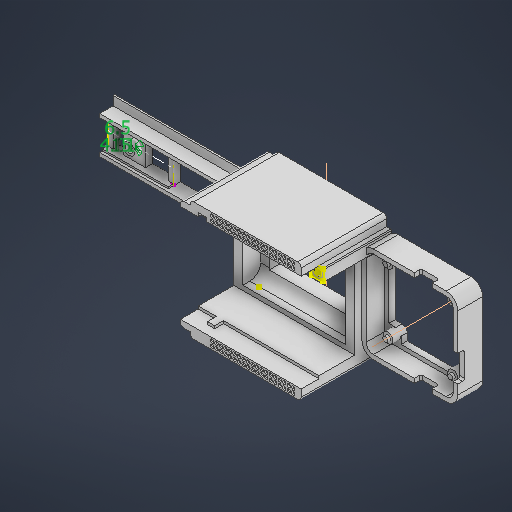
# Autodesk Inventor part: Base
Saved by Autodesk Inventor 2026 (Build 300175000, 175)
## iProperties
Created: 2026-08-27
Part Number: Base
Material: Generisch
Document SubType Name: Modeling
Designer: Fabian.Reifler
Density: 1 g/cm^3
Appearance: Vorgabe
Author: Fabian.Reifler
Autodesk Inventor part; units mm, degrees
sketch "Skizze1" plane through (0, 0, 0) normal (0, 0, 1) x (1, 0, 0)
  line L0 (-101.9645, 0) -> (106.7595, 0) construction
  line L1 (0, 139.1986) -> (0, -67.3687) construction
  line L2 (-143.7094, 0) -> (148.5043, 0) construction
  line L3 (0, -108.6821) -> (0, 180.5121) construction
  line L4 (-29, 23.45) -> (29, 23.45)
  line L5 (29, 23.45) -> (29, -23.45)
  line L6 (29, -23.45) -> (-29, -23.45)
  line L7 (-29, -23.45) -> (-29, 23.45)
  line L8 (-2.8134, 20.75) -> (4.8357, 20.75) construction
  line L9 (-2.8134, -20.75) -> (4.8357, -20.75) construction
  line L10 (-2.8134, 24.75) -> (4.8357, 24.75) construction
  line L11 (-2.8134, -24.75) -> (4.8357, -24.75) construction
  line L12 (-2.8134, 22.75) -> (5.1647, 22.75) construction
  circle A0 centre (0, 22.75) radius 2 construction
  circle A1 centre (0, -22.75) radius 2 construction
  line L13 (24, 18.45) -> (-24, 18.45)
  line L14 (-24, 18.45) -> (-24, -18.45)
  line L15 (-24, -18.45) -> (24, -18.45)
  line L16 (24, -18.45) -> (24, 18.45)
  line L17 (34, 28.45) -> (-34, 28.45)
  line L18 (-34, 28.45) -> (-34, -28.45)
  line L19 (-34, -28.45) -> (34, -28.45)
  line L20 (34, -28.45) -> (34, 28.45)
  line L21 (5, -40.2387) -> (5, 39.5986) construction
  line L22 (0, -22.75) -> (14.5212, -22.75) construction
  line L23 (0, 22.75) -> (17.4415, 22.75) construction
  point P0 (0, 0)
  point P1 (0, 24.75)
  point P2 (-1.8735, 23.45)
  point P3 (1.8735, 23.45)
  point P4 (5, 22.75)
  point P5 (5, -22.75)
  dimension "d0" = 58
  dimension "d1" = 46.9
  dimension "d2" = 41.5
  dimension "d3" = 4
  dimension "d4" = 5
  dimension "d5" = 5
  dimension "d79" = 10
  dimension "d104" = 5
  constraints: 44 end point, 10 point on line, 8 parallel, 7 horizontal, 4 perpendicular, 3 point on circle, 3 symmetric about line, 2 centre point, 2 collinear, 2 vertical, 1 coincident, 11 other
  measures "d0" distance of L4.start L4.end
  measures "d1" distance of L4.end L5.end
  measures "d2" distance between parallel lines of L9 L8
  measures "d3" distance between parallel lines of L10 L8
  measures "d4" distance between parallel lines of L4 L13
  measures "d5" distance between parallel lines of L4 L17
  measures "d79" diameter of L21 L3
  measures "d104" distance between parallel lines of L6 L15
extrude "Extrusion1" add sketch "Skizze1" along normal blind 8 contours L4 L5 L6 L7 | L16 L15 L14 L13 | L20 L19 L18 L17
extrude "Extrusion3" cut sketch "Skizze1" along normal through all contours L16 L15 L14 L13
hole "Bohrung1" at (5, -22.75, 0) at (5, 22.75, 0) direction (0, 0, 1) diameter 4.01 depth 6.5
sketch "Skizze2" plane through (0, 0, 8) normal (0, 0, 1) x (1, 0, 0)
  line L0 (29, 23.45) -> (29, -23.45) projected
  line L1 (29, -23.45) -> (-29, -23.45) projected
  line L2 (-29, 23.45) -> (29, 23.45) projected
  line L3 (-29, -23.45) -> (-29, 23.45) projected
  line L4 (-34, -28.45) -> (34, -28.45) projected
  line L5 (34, -28.45) -> (34, 28.45) projected
  line L6 (34, 28.45) -> (-34, 28.45) projected
  line L7 (-34, 28.45) -> (-34, -28.45) projected
  point P0 (0, 0)
extrude "Extrusion4" add sketch "Skizze2" along normal blind 10
fillet "Rundung1" radius 6 2 edges at (0, 23.45, 8) (0, -23.45, 8)
sketch "Skizze5" plane through (0, 0, 0) normal (0, 1, 0) x (-1, 0, 0)
  line L0 (-24, 8.0839) -> (24, 8.0839) projected
  line L1 (-31.8844, 48.0839) -> (73.7632, 48.0839)
  point P0 (0, 0)
  point P1 (0, 48.0839)
  dimension "d30" = 40
  constraints: 2 end point, 1 parallel, 1 point on line
  measures "d30" distance between parallel lines of L1 L0
ref_plane "Arbeitsebene6" through (0, 0, 48.0839) normal (0, 0, 1) x (1, 0, 0)
sketch "Skizze3" plane through (0, 0, 18) normal (0, 0, 1) x (1, 0, 0)
  line L0 (-34, 27.5) -> (34, 27.5)
  line L1 (34, 27.5) -> (34, -27.5)
  line L2 (34, -27.5) -> (-34, -27.5)
  line L3 (-34, -27.5) -> (-34, 27.5)
  line L4 (-95.3158, 0) -> (55.5526, 0) projected
  line L5 (0, -46.9) -> (0, 46.9) projected
  line L6 (-34, 27.5) -> (34, 27.5)
  line L7 (34, 27.5) -> (34, 33.5)
  line L8 (34, 33.5) -> (-34, 33.5)
  line L9 (-34, 33.5) -> (-34, 27.5)
  line L10 (-34, -27.5) -> (34, -27.5)
  line L11 (34, -27.5) -> (34, -33.5)
  line L12 (34, -33.5) -> (-34, -33.5)
  line L13 (-34, -33.5) -> (-34, -27.5)
  line L14 (34, -28.45) -> (34, 28.45) projected
  point P0 (0, 0)
  dimension "d22" = 55
  dimension "d24" = 6
  constraints: 24 end point, 4 parallel, 4 symmetric about line, 2 horizontal, 2 perpendicular, 1 collinear, 1 point on line, 2 other
  measures "d22" distance between parallel lines of L2 L0
  measures "d24" distance between parallel lines of L8 L0
extrude "Extrusion5" add sketch "Skizze3" along normal up to surface (30.0839 mm away) contours L9 L8 L5 L0 | L5 L8 L7 L0 | L2 L5 L12 L13 | L2 L11 L12 L5
sketch "Skizze4" plane through (0, 0, 18) normal (0, 0, -1) x (-1, 0, 0)
  line L0 (-34, 33.5) -> (34, 33.5) projected
  line L1 (34, 33.5) -> (34, 28.45) projected
  line L2 (-34, 28.45) -> (-34, 33.5) projected
  line L3 (-34, 28.45) -> (34, 28.45) projected
  line L4 (34, -33.5) -> (-34, -33.5) projected
  line L5 (34, -28.45) -> (34, -33.5) projected
  line L6 (-34, -33.5) -> (-34, -28.45) projected
  line L7 (34, -28.45) -> (-34, -28.45) projected
  point P0 (0, 0)
  point P1 (33.5, 28.45)
  point P2 (-33.5, 28.45)
  point P3 (33.5, -28.45)
  point P4 (-33.5, -28.45)
  constraints: 4 other
extrude "Extrusion6" add sketch "Skizze4" along normal up to surface (18 mm away)
fillet "Rundung2" radius 2 4 edges at (-34, -33.5, 24.042) (-34, 33.5, 24.042) (34, 33.5, 24.042) (34, -33.5, 24.042)
sketch "Skizze6" plane through (-34, 27.5, 48.0839) normal (0, 0, 1) x (1, 0, 0)
  line L0 (68, 0) -> (0, 0) projected
  line L1 (10, 0) -> (14.5, 0)
  line L2 (14.5, 0) -> (14.5, 2)
  line L3 (14.5, 2) -> (10, 2)
  line L4 (10, 2) -> (10, 0)
  line L5 (5, -50.95) -> (5, -4.05) projected
  point P0 (34, -27.5)
  dimension "d36" = 4.5
  dimension "d37" = 2
  dimension "d38" = 5
  constraints: 8 end point, 2 parallel, 1 horizontal, 1 perpendicular, 1 point on line
  measures "d36" distance of L2.end L3.end
  measures "d37" distance of L3.end L1.start
  measures "d38" distance between parallel lines of L5 L4
extrude "Extrusion7" cut sketch "Skizze6" against normal blind 10
sketch "Skizze7" plane through (-34, 27.5, 38.0839) normal (0, 0, 1) x (1, 0, 0)
  line L0 (10, 2) -> (14.5, 2) projected
  line L1 (12.25, 2) -> (12.25, -55) construction
  line L2 (0, -55) -> (68, -55) construction
  line L3 (14.25, -53.5) -> (10.25, -53.5)
  line L4 (10.25, -53.5) -> (10.25, -55)
  line L5 (10.25, -55) -> (14.25, -55)
  line L6 (14.25, -55) -> (14.25, -53.5)
  point P0 (34, -27.5)
  dimension "d41" = 4
  dimension "d42" = 1.5
  constraints: 10 end point, 2 parallel, 2 point on line, 1 horizontal, 1 midpoint, 1 perpendicular, 1 vertical, 1 other
  measures "d41" distance between parallel lines of L4 L6
  measures "d42" distance between parallel lines of L2 L3
extrude "Extrusion8" add sketch "Skizze7" along normal blind 5
sketch "Skizze8" plane through (0, 0, 0) normal (0, 0, 1) x (1, 0, 0)
  arc A0 (40.5, 24.5) -> (36.5, 20.5) centre (40.5, 20.5) ccw
  line L0 (36.5, 20.5) -> (36.5, -20.5)
  arc A1 (36.5, -20.5) -> (40.5, -24.5) centre (40.5, -20.5) ccw
  line L1 (40.5, -24.5) -> (81.5, -24.5)
  arc A2 (81.5, -24.5) -> (85.5, -20.5) centre (81.5, -20.5) ccw
  line L2 (85.5, -20.5) -> (85.5, 20.5)
  arc A3 (85.5, 20.5) -> (81.5, 24.5) centre (81.5, 20.5) ccw
  line L3 (81.5, 24.5) -> (40.5, 24.5)
  circle A4 centre (61, 0) radius 2.75
  circle A5 centre (79.25, 18.25) radius 3.25
  circle A6 centre (42.75, 18.25) radius 2.85
  circle A7 centre (42.75, -18.25) radius 2.85
  circle A8 centre (79.25, -18.25) radius 2.85
  circle A9 centre (42.75, -18.25) radius 1.4
  circle A10 centre (79.25, -18.25) radius 1.4
  circle A11 centre (79.25, 18.25) radius 1.4
  circle A12 centre (42.75, 18.25) radius 1.4
  line L4 (64.65, -27) -> (64.65, -24.5)
  line L5 (72.65, -27) -> (64.65, -27)
  line L6 (72.65, -24.5) -> (72.65, -27)
  line L7 (64.65, -24.5) -> (72.65, -24.5)
  line L8 (72.65, 27) -> (72.65, 24.5)
  line L9 (64.65, 27) -> (72.65, 27)
  line L10 (64.65, 24.5) -> (64.65, 27)
  line L11 (72.65, 24.5) -> (64.65, 24.5)
  line L12 (88, -14.15) -> (85.5, -14.15)
  line L13 (88, -1.15) -> (88, -14.15)
  line L14 (85.5, -1.15) -> (88, -1.15)
  line L15 (85.5, -14.15) -> (85.5, -1.15)
  line L16 (88, 20.5) -> (88, -20.5)
  arc A13 (81.5, -27) -> (88, -20.5) centre (81.5, -20.5) ccw
  line L17 (81.5, -27) -> (40.5, -27)
  arc A14 (34, -20.5) -> (40.5, -27) centre (40.5, -20.5) ccw
  line L18 (34, -20.5) -> (34, 20.5)
  arc A15 (40.5, 27) -> (34, 20.5) centre (40.5, 20.5) ccw
  line L19 (40.5, 27) -> (81.5, 27)
  arc A16 (88, 20.5) -> (81.5, 27) centre (81.5, 20.5) ccw
  line L20 (63.65, 24.5) -> (63.65, 27)
  line L21 (73.65, 27) -> (73.65, 24.5)
  line L22 (85.5, -0.15) -> (88, -0.15)
  line L23 (63.65, -27) -> (63.65, -24.5)
  line L24 (73.65, -24.5) -> (73.65, -27)
  line L25 (34, -26.45) -> (34, 26.45)
  line L26 (61, -31.4847) -> (61, 36.027) construction
  line L27 (79.25, 18.25) -> (42.75, 18.25) construction
  line L28 (42.75, 18.25) -> (42.75, -18.25) construction
  line L29 (42.75, -18.25) -> (79.25, -18.25) construction
  line L30 (79.25, -18.25) -> (79.25, 18.25) construction
  line L31 (0, -44.987) -> (0, 49.5293) construction
  line L32 (-107.4158, 0) -> (128.1526, 0) construction
  line L33 (81.5, -20.5) -> (40.5, -20.5) construction
  line L34 (40.5, -20.5) -> (40.5, 20.5) construction
  line L35 (40.5, 20.5) -> (81.5, 20.5) construction
  line L36 (81.5, 20.5) -> (81.5, -20.5) construction
  line L37 (88, -15.15) -> (85.5, -15.15)
  point P0 (81.65, 27)
  point P1 (94.5, -1.15)
  point P2 (94.5, -14.15)
  point P3 (81.65, -24.5)
  point P4 (73.65, -24.5)
  point P5 (73.65, 24.5)
  point P6 (81.65, 24.5)
  point P7 (81.65, 27)
  point P8 (88, -1.15)
  point P9 (72.65, -27)
  point P10 (0, 0)
  dimension "d49" = 2.5
  dimension "d50" = 2.8
  dimension "d51" = 2.8
  dimension "d52" = 2.8
  dimension "d53" = 2.8
  dimension "d129" = 36.5
  dimension "d133" = 24.5
  dimension "d134" = 24.5
  dimension "d135" = 24.5
  dimension "d138" = 2.5
  dimension "d140" = 54
  dimension "d141" = 5.5
  dimension "d142" = 6.5
  dimension "d143" = 6.5
  dimension "d144" = 6.5
  dimension "d145" = 6.5
  dimension "d153" = 36.5
  dimension "d154" = 36.5
  dimension "d157" = 36.5
  dimension "d158" = 36.5
  dimension "d159" = 5.7
  dimension "d160" = 5.7
  dimension "d161" = 5.7
  dimension "d162" = 6.5
  dimension "d163" = 41
  dimension "d164" = 41
  dimension "d165" = 36.5
  dimension "d166" = 41
  dimension "d167" = 1
  dimension "d168" = 1
  dimension "d169" = 5.3
  dimension "d174" = 1
  dimension "d175" = 1
  dimension "d176" = 8
  dimension "d178" = 8
  dimension "d181" = 2.5
  dimension "d182" = 41
  dimension "d185" = 13
  dimension "d188" = 1
  dimension "d189" = 5.3
  dimension "d191" = 54
  dimension "d192" = 34
  dimension "d193" = 1
  dimension "d194" = 3.1
  constraints: 72 end point, 25 centre point, 16 point on circle, 14 point on line, 11 perpendicular, 4 concentric, 2 collinear, 2 horizontal, 1 parallel, 1 vertical, 10 other
  measures "d49" distance between parallel lines of L3 L19
  measures "d50" diameter of A9
  measures "d51" diameter of A10
  measures "d52" diameter of A11
  measures "d53" diameter of A12
  measures "d129" distance of A7.centre A8.centre
  measures "d133" distance from line of L0 A4.centre
  measures "d134" distance from line of L2 A4.centre
  measures "d135" distance from line of L1 A4.centre
  measures "d138" distance between parallel lines of L17 L1
  measures "d140" distance between parallel lines of L19 L17
  measures "d141" diameter of A4
  measures "d142" radius of A13
  measures "d143" radius of A14
  measures "d144" radius of A15
  measures "d145" radius of A16
  measures "d153" diameter of L32 L27
  measures "d154" distance between parallel lines of L27 L29
  measures "d157" distance of L29.end L27.start
  measures "d158" diameter of A4.centre L28
  measures "d159" diameter of A8
  measures "d160" diameter of A7
  measures "d161" diameter of A6
  measures "d162" diameter of A5
  measures "d163" diameter of A4.centre L36
  measures "d164" distance between parallel lines of L33 L35
  measures "d165" diameter of A5.centre L26
  measures "d166" distance between parallel lines of L34 L36
  measures "d167" distance between parallel lines of L23 L4
  measures "d168" distance between parallel lines of L24 L6
  measures "d169" diameter of L23 L26
  measures "d174" distance between parallel lines of L20 L10
  measures "d175" distance between parallel lines of L8 L21
  measures "d176" distance between parallel lines of L10 L8
  measures "d178" distance between parallel lines of L4 L6
  measures "d181" distance between parallel lines of L18 L0
  measures "d182" distance of L2.start L2.end
  measures "d185" distance between parallel lines of L14 L12
  measures "d188" distance between parallel lines of L14 L22
  measures "d189" diameter of L20 L26
  measures "d191" diameter of L18 L26
  measures "d192" distance from line of L18 point (0, 0)
  measures "d193" distance between parallel lines of L37 L12
  measures "d194" distance between parallel lines of L37 L29
extrude "Boden" add sketch "Skizze8" along normal blind 3.5 contours L3 A3 L2 A2 L1 A1 L0 A0 | A0 L0 A1 L1 L23 L17 A14 L18 A15 L19 L20 L3 | L20 L19 L10 L3 | L10 L9 L8 L3 | L8 L19 L21 L3 | L1 L4 L17 L23 | L21 L19 A16 L16 L22 L2 A3 L3 | L1 L6 L5 L4 | L1 L24 L17 L6 | L1 A2 L2 L37 L16 A13 L17 L24 | L22 L16 L14 L2 | L14 L13 L12 L2 | L12 L16 L37 L2 | A4 | A5 | A6 | A7 | A8 | A9 | A10 | A11 | A12
extrude "ZapfenKlein" add sketch "Skizze8" along normal blind 9.5 contours A9 | A10 | A11 | A12
extrude "ZapfenGross" add sketch "Skizze8" along normal blind 8 contours A5 | A6 | A7 | A8 | A9 | A11 | A12
extrude "SteckerDurchführungen" add sketch "Skizze8" along normal blind 10.25 contours L20 L19 L10 L3 | L10 L9 L8 L3 | L8 L19 L21 L3 | L1 L4 L17 L23 | L1 L6 L5 L4 | L1 L24 L17 L6 | L22 L16 L14 L2 | L14 L13 L12 L2 | L12 L16 L37 L2
extrude "Extrusion18" add sketch "Skizze8" along normal blind 14 contours A0 L0 A1 L1 L23 L17 A14 L18 A15 L19 L20 L3 | L21 L19 A16 L16 L22 L2 A3 L3 | L1 A2 L2 L37 L16 A13 L17 L24
ref_plane "Arbeitsebene7" through (90.5, 27, 0) normal (0, 0, -1) x (-1, 0, 0)
fillet "Rundung4" radius 1 6 edges at (73.65, -25.75, 10.25) (86.75, -15.15, 10.25) (73.65, 25.75, 10.25) (86.75, -0.15, 10.25) (63.65, 25.75, 10.25) (63.65, -25.75, 10.25)
sketch "Skizze12" plane through (0, 0, 3.5) normal (0, 0, 1) x (1, 0, 0)
  circle A0 centre (42.75, 18.25) radius 2.85 projected
  circle A1 centre (79.25, 18.25) radius 3.25 projected
  circle A2 centre (79.25, -18.25) radius 2.85 projected
  circle A3 centre (42.75, -18.25) radius 2.85 projected
  line L0 (42.75, 15.4) -> (42.75, -15.4)
  line L1 (45.6, -18.25) -> (76.4, -18.25)
  line L2 (80.3336, -15.614) -> (80.3336, 15.186)
  line L3 (45.386, 17.1664) -> (76.186, 17.1664)
  point P0 (0, 0)
  dimension "d198" = 30.8
  dimension "d199" = 30.8
  dimension "d200" = 30.8
  dimension "d201" = 30.8
  constraints: 8 end point, 8 point on circle, 3 perpendicular, 1 horizontal, 1 vertical
  measures "d198" distance of L3.start L3.end
  measures "d199" distance of L2.start L2.end
  measures "d200" distance of L0.start L0.end
  measures "d201" distance of L1.start L1.end
extrude "Extrusion21" cut sketch "Skizze12" against normal through all contours A0 L3 A1 L2 A2 L1 A3 L0
sketch "Skizze13" plane through (-34, 0, 0) normal (-1, 0, 0) x (0, 0, 1)
  line L0 (0, 0) -> (18, 0) construction
  line L1 (0, 8.5) -> (8.5, 8.5)
  line L2 (0, 10.5) -> (8.5, 10.5)
  line L3 (8.5, 10.5) -> (8.5, 8.5)
  line L4 (0, 10.5) -> (0, 8.5) construction
  line L5 (0, -10.5) -> (8.5, -10.5)
  line L6 (8.5, -10.5) -> (8.5, -8.5)
  line L7 (0, -10.5) -> (0, -8.5) construction
  line L8 (0, 10.5) -> (0, 8.5)
  line L9 (0, -8.5) -> (0, -10.5)
  line L10 (0, 31.5) -> (0, -31.5) projected
  line L11 (8.5, -8.5) -> (0, -8.5)
  point P0 (8.5, -9.5)
  dimension "d203" = 2
  dimension "d311" = 8.5
  constraints: 22 end point, 4 symmetric about line, 3 perpendicular, 1 collinear, 1 midpoint
  measures "d203" distance between parallel lines of L2 L1
  measures "d311" distance between parallel lines of L10 L6
extrude "Extrusion22" add sketch "Skizze13" along normal blind 85
sketch "Skizze14" plane through (0, 0, 0) normal (0, 0, -1) x (-1, 0, 0)
  line L0 (119, 10.5) -> (119, 8.5)
  line L1 (119, 8.5) -> (82, 8.5)
  line L2 (82, 8.5) -> (82, -8.5)
  line L3 (82, -8.5) -> (119, -8.5)
  line L4 (119, -8.5) -> (119, 8.5)
  line L5 (119, -8.5) -> (119, -10.5) projected
  point P0 (0, 0)
  dimension "d207" = 37
  dimension "d312" = 17
  constraints: 10 end point, 2 collinear, 2 parallel, 1 horizontal, 1 perpendicular
  measures "d207" distance of L3.end L2.end
  measures "d312" distance of L3.end L0.end
extrude "Extrusion23" add sketch "Skizze14" against normal blind 4
sketch "Skizze15" plane through (0, 0, 4) normal (0, 0, 1) x (1, 0, 0)
  line L0 (-119, 8.5) -> (-119, -8.5) projected
  line L1 (-119, 0) -> (-82, 0) construction
  line L2 (-82, -8.5) -> (-82, 8.5) construction
  circle A0 centre (-104, 0) radius 3.25
  circle A1 centre (-104, 0) radius 2.005
  point P0 (0, 0)
  dimension "d210" = 15
  dimension "d218" = 6.5
  dimension "d219" = 4.01
  constraints: 2 centre point, 2 coincident, 2 end point, 2 midpoint, 1 point on line
  measures "d210" distance from line of L0 point (-104, 0)
  measures "d218" diameter of A0
  measures "d219" diameter of A1
extrude "Extrusion24" add sketch "Skizze15" along normal blind 3
sketch "Skizze17" plane through (79.25, 18.25, 9.5) normal (0, 0, 1) x (1, 0, 0)
  circle A0 centre (0, 0) radius 1.4 projected
  point P0 (-79.25, -18.25)
  constraints: 1 coincident
hole "Bohrung4" at (79.25, 18.25, 9.5) direction (0, 0, -1) diameter 4.01 depth 8
sketch "Skizze18" plane through (-104, 0, 7) normal (0, 0, 1) x (1, 0, 0)
  circle A0 centre (0, 0) radius 2.005 projected
  point P0 (104, 0)
  constraints: 1 coincident
hole "Bohrung5" at (-104, 0, 7) direction (0, 0, -1) diameter 4.01 depth 6.5
sketch "Skizze19" plane through (-34, -8.5, 8.5) normal (0, 1, 0) x (1, 0, 0)
  line L0 (-85, 1.5) -> (-48, 1.5)
  line L1 (-48, 4.5) -> (-48, 1.5)
  line L2 (-48, 4.5) -> (-85, 4.5) projected
  line L3 (-85, 0) -> (-85, 4.5) projected
  line L4 (-85, 1.5) -> (-85, 4.5)
  line L5 (-85, 4.5) -> (-48, 4.5)
  point P0 (34, 8.5)
  dimension "d241" = 37
  dimension "d313" = 3
  constraints: 8 end point, 2 equal length, 1 horizontal, 1 perpendicular
  measures "d241" distance of L0.start L0.end
  measures "d313" distance between parallel lines of L2 L0
extrude "Extrusion26" add sketch "Skizze19" along normal blind 1
mirror "Spiegeln1" about plane through (0, 0, 0) normal (0, 1, 0) of "Extrusion26"
sketch "Skizze20" plane through (-34, -27.5, 18) normal (0, 1, 0) x (1, 0, 0)
  line L0 (0, 0) -> (0, -30.0839) projected
  line L1 (0, -20.0839) -> (68, -20.0839)
  line L2 (68, 0) -> (68, -30.0839) projected
  line L3 (0, 0) -> (68, 0)
  line L4 (10.25, -25.0839) -> (10.25, -20.0839) projected
  line L5 (14.25, -25.0839) -> (10.25, -25.0839) projected
  line L6 (0, -20.0839) -> (0, 0)
  line L7 (68, -20.0839) -> (68, 0)
  line L8 (10.25, -20.0839) -> (14.25, -20.0839) projected
  line L9 (0, 0) -> (68, 0) projected
  point P0 (34, 18)
  dimension "d246" = 68
  constraints: 8 end point, 4 point on line, 3 collinear, 2 parallel, 2 perpendicular, 1 horizontal
  measures "d246" distance of L1.start L1.end
extrude "Extrusion27" add sketch "Skizze20" along normal up to surface (1.5 mm away)
mirror "Spiegeln2" about plane through (0, 0, 0) normal (0, 1, 0) of "Extrusion27"
sketch "Skizze22" plane through (-32, 33.5, 48.0839) normal (0, 0, 1) x (1, 0, 0)
  line L0 (10.75, 1.5) -> (10.75, -68.5) construction
  line L1 (10.75, -68.5) -> (93.25, -68.5) construction
  line L2 (93.25, -68.5) -> (93.25, 1.5) construction
  line L3 (93.25, 1.5) -> (10.75, 1.5) construction
  line L4 (10.75, 1.5) -> (93.25, -68.5) construction
  line L5 (10.75, -68.5) -> (93.25, 1.5) construction
  line L6 (93.25, -33.5) -> (10.75, -33.5) construction
  line L7 (68.29, 1.5) -> (68.29, -68.5) construction
  line L8 (68.29, -9.37) -> (10.75, -9.37) construction
  line L9 (68.29, -57.63) -> (10.75, -57.63) construction
  line L10 (10.75, -1.75) -> (93.25, -1.75) construction
  line L11 (10.75, -65.25) -> (93.25, -65.25) construction
  line L12 (-15.75, -4.29) -> (66.75, -4.29) construction
  line L13 (-15.75, -62.71) -> (66.75, -62.71) construction
  line L14 (3, -56.95) -> (3, -10.05) construction
  line L15 (-68.7658, -33.5) -> (120.2526, -33.5) projected
  line L16 (61, -10.05) -> (61, -56.95) projected
  line L17 (32, -82.5) -> (32, 15.5) projected
  line L18 (-68.7658, -33.5) -> (120.2526, -33.5) projected
  line L19 (51.35, -4.29) -> (51.35, -14.1898) construction
  line L20 (68.82, -5.87) -> (68.82, -12.87)
  line L21 (68.82, -12.87) -> (61.82, -12.87)
  line L22 (61.82, -12.87) -> (61.82, -5.87)
  line L23 (61.82, -5.87) -> (68.82, -5.87)
  line L24 (68.82, -5.87) -> (61.82, -12.87) construction
  line L25 (68.82, -12.87) -> (61.82, -5.87) construction
  point P0 (52, -33.5)
  point P1 (15.79, -1.75)
  point P2 (15.79, -65.25)
  point P3 (18.33, -1.75)
  point P4 (20.87, -1.75)
  point P5 (23.41, -1.75)
  point P6 (25.95, -1.75)
  point P7 (28.49, -1.75)
  point P8 (31.03, -1.75)
  point P9 (33.57, -1.75)
  point P10 (36.11, -1.75)
  point P11 (38.65, -1.75)
  point P12 (41.19, -1.75)
  point P13 (43.73, -1.75)
  point P14 (46.27, -1.75)
  point P15 (48.81, -1.75)
  point P16 (51.35, -1.75)
  point P17 (53.89, -1.75)
  point P18 (56.43, -1.75)
  point P19 (58.97, -1.75)
  point P20 (61.51, -1.75)
  point P21 (15.79, -4.29)
  point P22 (18.33, -4.29)
  point P23 (20.87, -4.29)
  point P24 (23.41, -4.29)
  point P25 (25.95, -4.29)
  point P26 (28.49, -4.29)
  point P27 (31.03, -4.29)
  point P28 (33.57, -4.29)
  point P29 (36.11, -4.29)
  point P30 (38.65, -4.29)
  point P31 (41.19, -4.29)
  point P32 (43.73, -4.29)
  point P33 (46.27, -4.29)
  point P34 (48.81, -4.29)
  point P35 (53.89, -4.29)
  point P36 (56.43, -4.29)
  point P37 (58.97, -4.29)
  point P38 (61.51, -4.29)
  point P39 (18.33, -65.25)
  point P40 (20.87, -65.25)
  point P41 (23.41, -65.25)
  point P42 (25.95, -65.25)
  point P43 (28.49, -65.25)
  point P44 (31.03, -65.25)
  point P45 (33.57, -65.25)
  point P46 (36.11, -65.25)
  point P47 (38.65, -65.25)
  point P48 (41.19, -65.25)
  point P49 (43.73, -65.25)
  point P50 (46.27, -65.25)
  point P51 (48.81, -65.25)
  point P52 (51.35, -65.25)
  point P53 (53.89, -65.25)
  point P54 (56.43, -65.25)
  point P55 (58.97, -65.25)
  point P56 (61.51, -65.25)
  point P57 (15.79, -62.71)
  point P58 (18.33, -62.71)
  point P59 (20.87, -62.71)
  point P60 (23.41, -62.71)
  point P61 (25.95, -62.71)
  point P62 (28.49, -62.71)
  point P63 (31.03, -62.71)
  point P64 (33.57, -62.71)
  point P65 (36.11, -62.71)
  point P66 (38.65, -62.71)
  point P67 (41.19, -62.71)
  point P68 (43.73, -62.71)
  point P69 (46.27, -62.71)
  point P70 (48.81, -62.71)
  point P71 (51.35, -62.71)
  point P72 (53.89, -62.71)
  point P73 (56.43, -62.71)
  point P74 (58.97, -62.71)
  point P75 (61.51, -62.71)
  point P76 (52, -33.5)
  point P77 (52, -33.5)
  point P78 (32, -33.5)
  point P79 (52, -33.5)
  point P80 (65.32, -9.37)
  dimension "d251" = 82.5
  dimension "d252" = 70
  dimension "d254" = 57.54
  dimension "d257" = 63.5
  dimension "d258" = 48.26
  dimension "d259" = 5.04
  dimension "d260" = 2.54
  dimension "d261" = 2.54
  dimension "d264" = 2.54
  dimension "d271" = 2.54
  dimension "d278" = 2.54
  dimension "d285" = 2.54
  dimension "d292" = 2.54
  dimension "d299" = 2.54
  dimension "d307" = 20
  dimension "d321" = 13.97
  dimension "d322" = 7
  dimension "d323" = 7
  constraints: 42 end point, 10 midpoint, 8 point on line, 6 parallel, 5 perpendicular, 5 symmetric about line, 5 vertical, 4 horizontal, 1 collinear, 76 other
  measures "d251" distance of L0.end L1.end
  measures "d252" distance between parallel lines of L1 L3
  measures "d254" distance between parallel lines of L0 L7
  measures "d257" distance between parallel lines of L11 L10
  measures "d258" distance between parallel lines of L9 L8
  measures "d259" distance from line of point (15.79, -1.75) L0
  measures "d260" distance between parallel lines of L10 L12
  measures "d261" distance between parallel lines of L11 L13
  measures "d264" distance of point (15.79, -1.75) point (18.33, -1.75)
  measures "d271" distance of point (15.79, -1.75) point (15.79, -4.29)
  measures "d278" distance of point (15.79, -4.29) point (18.33, -4.29)
  measures "d285" distance of point (15.79, -65.25) point (18.33, -65.25)
  measures "d292" distance of point (15.79, -65.25) point (15.79, -62.71)
  measures "d299" distance of point (15.79, -62.71) point (18.33, -62.71)
  measures "d307" distance from line of point (52, -33.5) L17
  measures "d321" distance from line of L19 point (65.32, -9.37)
  measures "d322" distance of L20.end L21.end
  measures "d323" distance of L20.start L20.end
hole "Bohrung6" at (-16.21, 31.75, 48.0839) at (-13.67, 31.75, 48.0839) at (-13.67, 29.21, 48.0839) at (-16.21, 29.21, 48.0839) at (-11.13, 31.75, 48.0839) at (-8.59, 31.75, 48.0839) at (-6.05, 31.75, 48.0839) at (-3.51, 31.75, 48.0839) at (-0.97, 31.75, 48.0839) at (1.57, 31.75, 48.0839) at (29.51, 29.21, 48.0839) at (29.51, 31.75, 48.0839) at (26.97, 31.75, 48.0839) at (26.97, 29.21, 48.0839) at (24.43, 29.21, 48.0839) at (24.43, 31.75, 48.0839) at (21.89, 29.21, 48.0839) at (21.89, 31.75, 48.0839) at (19.35, 29.21, 48.0839) at (19.35, 31.75, 48.0839) at (16.81, 29.21, 48.0839) at (16.81, 31.75, 48.0839) at (14.27, 29.21, 48.0839) at (14.27, 31.75, 48.0839) at (11.73, 31.75, 48.0839) at (11.73, 29.21, 48.0839) at (9.19, 29.21, 48.0839) at (9.19, 31.75, 48.0839) at (6.65, 29.21, 48.0839) at (6.65, 31.75, 48.0839) at (4.11, 29.21, 48.0839) at (4.11, 31.75, 48.0839) at (1.57, 29.21, 48.0839) at (-0.97, 29.21, 48.0839) at (-3.51, 29.21, 48.0839) at (-6.05, 29.21, 48.0839) at (-8.59, 29.21, 48.0839) at (-11.13, 29.21, 48.0839) direction (0, 0, -1) diameter 1.5 depth 10 countersink diameter 2 countersink angle 45
mirror "Spiegeln3" about plane through (0, 0, 0) normal (0, 1, 0) of "Bohrung6"
extrude "Extrusion29" add sketch "Skizze22" against normal up to surface (48.0839 mm away)
fillet "Rundung6" radius 0.5 3 edges at (36.82, 27.63, 24.042) (36.82, 20.63, 25.792) (29.82, 20.63, 33.042)
hole "Bohrung7" at (33.32, 24.13, 48.0839) direction (0, 0, -1) diameter 4.01 depth 16.5
ref_plane "Arbeitsebene8" through (29.82, 26, 38.0839) normal (0, 0, 1) x (1, 0, 0)
sketch "Skizze25" plane through (29.82, 26, 38.0839) normal (0, 0, 1) x (1, 0, 0)
  arc A0 (7, 1.13) -> (6.5, 1.63) centre (6.5, 1.13) ccw projected
  line L0 (7, -4.87) -> (7, 1.13) projected
  arc A1 (6.5, -5.37) -> (7, -4.87) centre (6.5, -4.87) ccw projected
  arc A2 (0, -4.87) -> (0.5, -5.37) centre (0.5, -4.87) ccw projected
  line L1 (0, 1.5) -> (0, -4.87) projected
  line L2 (6.5, 1.63) -> (4.18, 1.63) projected
  line L3 (0.5, -5.37) -> (6.5, -5.37) projected
  line L4 (0, 1.5) -> (4.18, 1.5)
  line L5 (4.18, 1.5) -> (4.18, 1.63)
  circle A3 centre (3.5, -1.87) radius 2.005 projected
  point P0 (-29.82, -26)
  constraints: 4 end point, 1 parallel, 1 perpendicular
extrude "Extrusion30" cut sketch "Skizze25" along normal blind 10
extrude "Extrusion31" add sketch "Skizze25" along normal blind 10 separate body
sketch "Skizze27" plane through (0, 0, 4) normal (0, 0, 1) x (1, 0, 0)
  circle A0 centre (-104, 0) radius 3.25 projected
  line L0 (-82, 7.5) -> (-119, 7.5) projected
  line L1 (-119, 7.5) -> (-119, -7.5) projected
  line L2 (-119, -7.5) -> (-82, -7.5) projected
  line L3 (-82, -7.5) -> (-82, 7.5) projected
  line L4 (-85, 7.5) -> (-97.75, 7.5)
  line L5 (-97.75, 7.5) -> (-97.75, -7.5)
  line L6 (-97.75, -7.5) -> (-85, -7.5)
  line L7 (-85, -7.5) -> (-85, 7.5)
  line L8 (-110.25, 7.5) -> (-116, 7.5)
  line L9 (-116, 7.5) -> (-116, -7.5)
  line L10 (-116, -7.5) -> (-110.25, -7.5)
  line L11 (-110.25, -7.5) -> (-110.25, 7.5)
  line L12 (-119, -7.5) -> (-82, -7.5) projected
  point P0 (0, 0)
  point P1 (-116, -7.5)
  point P2 (-97.75, 7.5)
  dimension "d339" = 3
  dimension "d340" = 3
  dimension "d341" = 3
  dimension "d342" = 3
  constraints: 16 end point, 4 parallel, 3 point on line, 2 horizontal, 2 perpendicular, 1 collinear
  measures "d339" distance between parallel lines of L9 L1
  measures "d340" distance between parallel lines of L3 L7
  measures "d341" distance edge to line of A0 L5
  measures "d342" distance edge to line of A0 L11
extrude "Extrusion32" cut sketch "Skizze27" against normal through all contours L7 L2 L5 L0 | L11 L2 L9 L0
thicken "Verdickung1" operation cut thickness 4 both sides no extend neighbours no toward (0, 1, 0) faces at (65.9193, 17.1664, 2.3333)
thicken "Verdickung2" operation cut thickness 4 both sides no extend neighbours no toward (0, -1, 0) faces at (55.8667, -18.25, 2.3333)
thicken "Verdickung3" operation cut thickness 4 both sides no extend neighbours no toward (-1, 0, 0) faces at (42.75, 5.1333, 2.3333)
thicken "Verdickung4" operation cut thickness 4 both sides no extend neighbours no toward (1, 0, 0) faces at (80.3336, -5.3474, 2.3333)
sketch "Skizze28" plane through (-34, -10.5, 0) normal (0, -1, 0) x (1, 0, 0)
  line L0 (0, 0) -> (-85, 0) projected
  line L1 (-85, 0) -> (-85, 8.5) projected
  line L2 (0, 0) -> (-85, 0)
  line L3 (-85, 0) -> (-85, 1)
  line L4 (-85, 1) -> (0, 1)
  line L5 (0, 1) -> (0, 0)
  point P0 (34, 0)
  dimension "d354" = 1
  constraints: 8 end point, 2 parallel, 1 horizontal, 1 perpendicular, 1 point on line
  measures "d354" distance between parallel lines of L0 L4
extrude "Extrusion33" add sketch "Skizze28" along normal blind 5
mirror "Spiegeln4" about plane through (0, 0, 0) normal (0, 1, 0) of "Extrusion33"
sketch "Skizze29" plane through (-34, -27.5, 48.0839) normal (0, 0, 1) x (1, 0, 0)
  line L0 (0, -6) -> (5.5, -6)
  line L1 (5.5, -6) -> (5.5, -3.4)
  line L2 (5.5, -3.4) -> (0, -3.4)
  line L3 (0, -3.4) -> (0, -6)
  line L4 (34, 27.5) -> (-22.8526, 27.5) construction
  line L5 (0, 61) -> (5.5, 61)
  line L6 (5.5, 61) -> (5.5, 58.4)
  line L7 (5.5, 58.4) -> (0, 58.4)
  line L8 (0, 58.4) -> (0, 61)
  line L9 (66, -6) -> (2, -6) projected
  line L10 (0, -4) -> (0, 0) projected
  dimension "d357" = 61.8
  dimension "d358" = 5.5
  constraints: 18 end point, 4 symmetric about line, 2 collinear, 2 horizontal, 2 parallel, 1 perpendicular
  measures "d357" distance between parallel lines of L7 L2
  measures "d358" distance between parallel lines of L3 L1
extrude "Extrusion34" cut sketch "Skizze29" against normal through all
fillet "Rundung8" radius 2 4 edges at (-34, 30.9, 24.042) (-34, -30.9, 24.042) (-28.5, 33.5, 24.042) (-28.5, -33.5, 24.042)
